Autodesk Fusion 360 part; units mm, degrees
(part 2 of 2)
sketch "Esquisse15" plane through (0, 0, 0) normal (0, 0, 1) x (1, 0, 0)
  circle A0 centre (0, 500) radius 72.5
  circle A1 centre (0, 500) radius 69.5
  circle A2 centre (0, 500) radius 15
  line L0 (0, 485) -> (0, 486)
  circle A3 centre (0, 488.5) radius 2.5
  circle A4 centre (11.5, 500) radius 2.5
  circle A5 centre (0, 511.5) radius 2.5
  circle A6 centre (-11.5, 500) radius 2.5
  circle A7 centre (0, 625) radius 2.5
  circle A8 centre (0, 625) radius 3
  circle A9 centre (0, 500) radius 3
  dimension "d221" = 145
  dimension "d222" = -3
  dimension "d223" = 30
  dimension "d224" = 1
  dimension "d225" = 5
  dimension "d227" = 360
  dimension "d228" = 5
  dimension "d229" = 6
  dimension "d256" = 6
  constraint concentric A0 A2
  constraint coincident A2 L0.start
  constraint vertical L0
  constraint coincident L0.end A3
  constraint concentric A7 A8
  constraint concentric A0 A9
  measures "d221" diameter of A0
  measures "d223" diameter of A2
  measures "d224" distance of L0.start L0.end
  measures "d225" diameter of A3
  measures "d228" diameter of A7
  measures "d229" diameter of A8
  measures "d256" diameter of A9
extrude "Extrusion40" add sketch "Esquisse15" along normal blind 16 separate body contours A7 picked at (-0.185434, 625.81244) makes body 74
extrude "Extrusion41" add sketch "Esquisse15" along normal blind 0.6 separate body contours A8 picked at (-2.478015, 626.358774) makes body 75
move_body "Déplacer26" bodies 75 to x (1, 0, 0) y (0, 1, 0) z (0, 0, 1) at (0, 0, 7.7)
combine "Combiner11" operation add target body 74 tool bodies 75
move_body "Déplacer27" bodies 74 to x (1, 0, 0) y (0, 1, 0) z (0, 0, 1) at (-11.5, -125, 0)
move_body "Déplacer28" bodies 74 to x (1, 0, 0) y (0, 1, 0) z (0, 0, 1) at (0, 0, 3)
pattern_circular "Réseau C3" count 4 over 360 about axis through (0, 500, 0) along (0, 0, 1) of bodies 74 makes body 76 at (-2.462019, 488.93412, 5.566667) makes body 77 at (13.415111, 501.606969, 8.133333) makes body 78 at (2.480598, 511.810859, 5.566667)
extrude "Extrusion42" add sketch "Esquisse15" along normal blind 9 separate body contours A1 | A2 | A3 | A4 | A5 | A6 | A9 picked at (0, 448.796224) picked at (-7.340893, 492.306801) picked at (0.209792, 490.067641) picked at (11.195549, 500.775728) picked at (0.185434, 510.760984) picked at (-11.804451, 500.775728) picked at (-0.826239, 499.138595) makes body 79
combine "Combiner12" operation cut target body 79 tool bodies 77 78 74 76 keep tools
extrude "Extrusion43" add sketch "Esquisse15" along normal blind 8 separate body contours A1 | A2 | A9 picked at (0, 448.796224) picked at (-7.340893, 492.306801) picked at (-0.826239, 499.138595) makes body 80
move_body "Déplacer29" bodies 80 to x (1, 0, 0) y (0, 1, 0) z (0, 0, 1) at (0, 0, 12)
sketch "Esquisse16" plane through (0, 0, 0) normal (0, 0, 1) x (1, 0, 0)
  line L0 (-27.886751, 605) -> (-30.773503, 600)
  line L1 (-30.773503, 600) -> (-27.886751, 595)
  line L2 (-27.886751, 595) -> (-22.113249, 595)
  line L3 (-22.113249, 595) -> (-19.226497, 600)
  line L4 (-19.226497, 600) -> (-22.113249, 605)
  line L5 (-22.113249, 605) -> (-27.886751, 605)
  circle A0 centre (-75, 600) radius 6
  point P0 (-25, 600)
  dimension "d250" = 5
  dimension "d284" = 12
  measures "d250" distance of P0 L5
  measures "d284" diameter of A0
extrude "Extrusion44" add sketch "Esquisse16" along normal blind 6 separate body contours L0 L1 L2 L3 L4 L5 picked at (-25.96225, 598.333333) makes body 81
move_body "Déplacer30" bodies 81 to x (1, 0, 0) y (0, 1, 0) z (0, 0, 1) at (25, -100, 0)
combine "Combiner13" operation cut target body 79 tool bodies 81
extrude "Extrusion45" cut sketch "Esquisse15" along normal blind 50 contours A9 picked at (-0.826239, 499.138595) bodies 79 80
copy_body "Copier/Coller des corps10" bodies 80 makes body 82
move_body "Déplacer32" bodies 82 to x (1, 0, 0) y (0, 1, 0) z (0, 0, 1) at (0, 190, 0)
extrude "Extrusion46" add sketch "Esquisse16" along normal blind 5 separate body contours L0 L1 L2 L3 L4 L5 picked at (-25.96225, 598.333333) makes body 83
move_body "Déplacer33" bodies 83 to x (1, 0, 0) y (0, 1, 0) z (0, 0, 1) at (25, -100, 0)
move_body "Déplacer34" bodies 83 to x (1, 0, 0) y (0, 1, 0) z (0, 0, 1) at (0, 0, 15)
sketch "Esquisse17" plane through (0, 0, 0) normal (0, 0, 1) x (1, 0, 0)
  circle A0 centre (-25, 600) radius 5.95
  point P0 (-25, 600)
  dimension "d267" = 11.9
  constraint coincident P0 A0.centre
  measures "d267" diameter of A0
extrude "Extrusion47" add sketch "Esquisse17" along normal blind 5 separate body contours A0 picked at (-25.441333, 601.933607) makes body 84
move_body "Déplacer35" bodies 84 to x (1, 0, 0) y (0, 1, 0) z (0, 0, 1) at (25, -100, 0)
move_body "Déplacer36" bodies 84 to x (1, 0, 0) y (0, 1, 0) z (0, 0, 1) at (0, 0, 15)
combine "Combiner14" operation cut target body 80 tool bodies 84
extrude "Extrusion48" add sketch "Esquisse15" along normal blind 16 separate body contours A1 | A2 | A3 | A4 | A5 | A6 | A9 picked at (0, 448.796224) picked at (-7.340893, 492.306801) picked at (0.209792, 490.067641) picked at (11.195549, 500.775728) picked at (0.185434, 510.760984) picked at (-11.804451, 500.775728) picked at (-0.826239, 499.138595) makes body 85
move_body "Déplacer37" bodies 85 to x (1, 0, 0) y (0, 1, 0) z (0, 0, 1) at (0, 0, 12)
combine "Combiner15" operation cut target body 85 tool bodies 80 keep tools
move_body "Déplacer38" bodies 85 to x (1, 0, 0) y (0, 1, 0) z (0, 0, 1) at (0, 0, 60)
move_body "Déplacer39" bodies 80 to x (1, 0, 0) y (0, 1, 0) z (0, 0, 1) at (0, 0, 15)
sketch "Esquisse18" plane through (0, 0, 0) normal (0, 0, 1) x (1, 0, 0)
  circle A0 through (-22, 600.000002, 0.000749) (-26.499998, 602.598028, -0.015936) (-26.500002, 597.401969, 0.015187)
  line L0 (-25.153205, 602.996032, -0.017983) -> (-25.153205, 606.000009, -0.017983) construction
  point P0 (-25, 600)
  dimension "d285" = 6
extrude "Extrusion49" add sketch "Esquisse18" along normal blind 3.6 separate body contours A0 in plane through (-0.000898, 0.021562, 3.599871) normal (-0.00024956, 0.00598949, 0.99998203) picked at (-24.417479, 598.029913, 0.011945) makes body 86
sketch "Esquisse19" plane through (-0.001797, 0.043124, 7.199806) normal (-0.00024956, 0.00598949, 0.99998203) x (-0.99913307, -0.04163054, 0)
  circle A0 centre (0, -600.509817) radius 3
  circle A1 centre (0, -600.509817) radius 3
  constraint concentric A0 A1
loft "Lissage1" add profiles "Esquisse17", "Esquisse19" section 1 contours A0 picked at (-25.441333, 601.933607) section 2 contours A0 A1 picked at (1.068532, -599.727986) bodies 86
extrude "Extrusion50" add sketch "Esquisse18" along normal blind 25 contours A0 in plane through (-0.000898, 0.021562, 3.599871) normal (-0.00024956, 0.00598949, 0.99998203) picked at (-24.417479, 598.029913, 0.011945) bodies 86
move_body "Déplacer40" bodies 86 to x (-1, 0, 0) y (0, 1, 0) z (0, 0, -1) at (-50.30641, 0, -0.035967)
copy_body "Copier/Coller des corps11" bodies 86 makes body 87
move_body "Déplacer41" bodies 87 to x (1, 0, 0) y (0, 1, 0) z (0, 0, 1) at (25, -100, 0)
extrude "Extrusion51" add sketch "Esquisse15" along normal blind 3.5 separate body contours A1 | A2 | A3 | A4 | A5 | A6 | A9 picked at (0, 448.796224) picked at (-7.340893, 492.306801) picked at (0.209792, 490.067641) picked at (11.195549, 500.775728) picked at (0.185434, 510.760984) picked at (-11.804451, 500.775728) picked at (-0.826239, 499.138595) makes body 88
move_body "Déplacer42" bodies 88 to x (1, 0, 0) y (0, 1, 0) z (0, 0, 1) at (0, 0, 17.5)
move_body "Déplacer43" bodies 87 to x (1, 0, 0) y (0, 1, 0) z (0, 0, 1) at (0, 0, 21.2)
combine "Combiner16" operation cut target body 88 tool bodies 87 keep tools
combine "Combiner17" operation cut target body 88 tool bodies 78 77 76 74 keep tools
extrude "Extrusion52" add sketch "Esquisse15" along normal blind 4 separate body contours A2 picked at (-7.340893, 492.306801) makes body 89
move_body "Déplacer44" bodies 89 to x (1, 0, 0) y (0, 1, 0) z (0, 0, 1) at (0, 0, 7.25)
combine "Combiner18" operation add target body 89 tool bodies 79 keep tools
combine "Combiner19" operation cut target body 79 tool bodies 78 74 77 76 keep tools
copy_body "Copier/Coller des corps12" bodies 87 74 78 77 76 makes body 90 makes body 91 makes body 92 makes body 93 makes body 94
move_body "Déplacer45" bodies 90 91 92 93 94 to x (1, 0, 0) y (0, 1, 0) z (0, 0, 1) at (-390, 90, 0)
sketch "Esquisse20" plane through (0, 0, 0) normal (0, 0, 1) x (1, 0, 0)
  circle A0 centre (-390.000006, 590.000009) radius 25
  circle A1 centre (-390.000006, 590.000009) radius 50
  circle A2 centre (-390, 590) radius 100
  dimension "d307" = 50
  dimension "d308" = 100
  dimension "d309" = 200
  constraint concentric A0 A1
  measures "d307" diameter of A0
  measures "d308" diameter of A1
  measures "d309" diameter of A2
move_body "Déplacer46" bodies 93 94 92 90 91 to x (1, 0, 0) y (0, 1, 0) z (0, 0, 1) at (0, 0, -18)
move_body "Déplacer47" bodies 93 94 91 92 to x (1, 0, 0) y (0, 1, 0) z (0, 0, 1) at (0, 0, 2.3)
extrude "Extrusion53" add sketch "Esquisse20" along normal blind 3 separate body contours A0 picked at (-383.89124, 598.152153) makes body 95
extrude "Extrusion54" add sketch "Esquisse20" along normal blind 3 separate body contours A0 | A1 picked at (-383.89124, 598.152153) picked at (-348.612568, 586.273952) makes body 96
extrude "Extrusion55" add sketch "Esquisse20" along normal blind 3 separate body contours A0 | A1 | A2 picked at (-383.89124, 598.152153) picked at (-348.612568, 586.273952) picked at (-376.382952, 508.013481) makes body 97
combine "Combiner20" operation cut target body 95 tool bodies 94 93 92 90 91 keep tools
combine "Combiner21" operation cut target body 96 tool bodies 94 92 91 93 90 keep tools
combine "Combiner22" operation cut target body 97 tool bodies 94 90 93 91 92 keep tools
move_body "Déplacer48" bodies 97 to x (1, 0, 0) y (0, 1, 0) z (0, 0, 1) at (0, 220, 0)
move_body "Déplacer49" bodies 96 to x (1, 0, 0) y (0, 1, 0) z (0, 0, 1) at (-170, 0, 0)
move_body "Déplacer50" bodies 95 to x (1, 0, 0) y (0, 1, 0) z (0, 0, 1) at (0, -160, 0)
sketch "Esquisse21" plane through (0, 0, 0) normal (0, 0, 1) x (1, 0, 0)
  circle A0 centre (-390.000006, 590.000009) radius 15
  line L0 (-404.500006, 590.000009) -> (-405.000006, 590.000009)
  circle A1 centre (-401.500006, 590.000009) radius 3
  circle A2 centre (-390.000006, 578.500009) radius 3
  circle A3 centre (-378.500006, 590.000009) radius 3
  circle A4 centre (-390.000006, 601.500009) radius 3
  circle A5 centre (-390.000006, 590.000009) radius 3
  circle A6 centre (-390.000006, 590.000009) radius 35
  dimension "d331" = 30
  dimension "d334" = 6
  dimension "d336" = 360
  dimension "d337" = 6
  dimension "d338" = 70
  constraint horizontal L0
  constraint concentric A0 A5
  constraint concentric A5 A6
  measures "d331" diameter of A0
  measures "d334" diameter of A1
  measures "d337" diameter of A5
  measures "d338" diameter of A6
extrude "Extrusion57" add sketch "Esquisse21" along normal blind 2 separate body contours A0 | A6 picked at (-382.175174, 597.536911) picked at (-361.852825, 587.515971) makes body 98
extrude "Extrusion56" add sketch "Esquisse21" against normal blind 3 separate body contours A0 picked at (-382.175174, 597.536911) makes body 99
move_body "Déplacer51" bodies 98 to x (1, 0, 0) y (0, 1, 0) z (0, 0, 1) at (0, 0, -5)
combine "Combiner23" operation add target body 98 tool bodies 99 keep tools
extrude "Extrusion58" add sketch "Esquisse21" against normal blind 22 separate body contours A0 | A1 | A2 | A3 | A4 | A6 picked at (-382.175174, 597.536911) picked at (-402.854178, 589.218177) picked at (-391.354178, 577.718177) picked at (-379.014807, 589.069135) picked at (-390.514807, 600.569135) picked at (-361.852825, 587.515971) makes body 100
extrude "Extrusion59" add sketch "Esquisse21" against normal blind 5 separate body contours A0 | A1 | A2 | A3 | A4 | A5 | A6 picked at (-382.175174, 597.536911) picked at (-402.854178, 589.218177) picked at (-391.354178, 577.718177) picked at (-379.014807, 589.069135) picked at (-390.514807, 600.569135) picked at (-390.623496, 591.371351) picked at (-361.852825, 587.515971) makes body 101
combine "Combiner24" operation cut target body 100 tool bodies 101
combine "Combiner25" operation add target body 99 tool bodies 98
extrude "Extrusion60" cut sketch "Esquisse21" against normal blind 14 contours A1 | A2 | A3 | A4 picked at (-402.854178, 589.218177) picked at (-391.354178, 577.718177) picked at (-379.014807, 589.069135) picked at (-390.514807, 600.569135) bodies 100
copy_body "Copier/Coller des corps13" bodies 100 makes body 102
move_body "Déplacer52" bodies 102 to x (1, 0, 0) y (0, 1, 0) z (0, 0, 1) at (85, 0, 0)
extrude "Extrusion61" add sketch "Esquisse16" along normal blind 10 separate body contours L0 L1 L2 L3 L4 L5 picked at (-25.96225, 598.333333) makes body 103
move_body "Déplacer53" bodies 103 to x (1, 0, 0) y (0, 1, 0) z (0, 0, 1) at (-280.000006, -9.999991, -5)
move_body "Déplacer54" bodies 103 to x (1, 0, 0) y (0, 1, 0) z (0, 0, 1) at (0, 0, -10)
combine "Combiner26" operation cut target body 102 tool bodies 103
move_body "Déplacer55" bodies 100 to x (1, 0, 0) y (0, 1, 0) z (0, 0, 1) at (0, -90, 0)
copy_body "Copier/Coller des corps14" bodies 99 makes body 104
move_body "Déplacer56" bodies 104 to x (1, 0, 0) y (0, 1, 0) z (0, 0, 1) at (85, 0, 10)
extrude "Extrusion62" add sketch "Esquisse21" along normal blind 4 separate body contours A0 picked at (-382.175174, 597.536911) makes body 105
move_body "Déplacer57" bodies 105 to x (1, 0, 0) y (0, 1, 0) z (0, 0, 1) at (-110, -70, 0)
component "Spur Gear (16 teeth)" placed x (1, 0, 0) y (0, 1, 0) z (0, 0, 1) at (0, 0, 0)
equation "BaseHeight = 8 mm"
equation "d15 = BaseHeight"
equation "d21 = BaseHeight / 2"
equation "d23 = BaseHeight / 2"
equation "d29 = BaseHeight / 2"
equation "d33 = BaseHeight * 2"
equation "d54 = BaseHeight"
equation "d93 = ( 40 * 2 ) * 1 mm"
equation "d172 = BaseHeight + 1 mm"
equation "d190 = BaseHeight"
equation "d194 = BaseHeight"
equation "d195 = BaseHeight"
equation "d200 = 3 mm + BaseHeight"
equation "d202 = BaseHeight + 3 mm"
equation "d207 = BaseHeight"
equation "d230 = MetalHeight"
equation "d236 = 8 mm - 0.3 mm"
equation "MetalHeight = 16 mm"
equation "d243 = 3 mm + MetalHeight / 2 - 2 mm"
equation "d245 = MetalHeight / 2"
equation "d249 = MetalHeight / 2 + 4 mm"
equation "d273 = MetalHeight"
equation "d295 = 19.00 mm - 1.5 mm"
equation "d303 = 8.00 mm - 0.75 mm"
